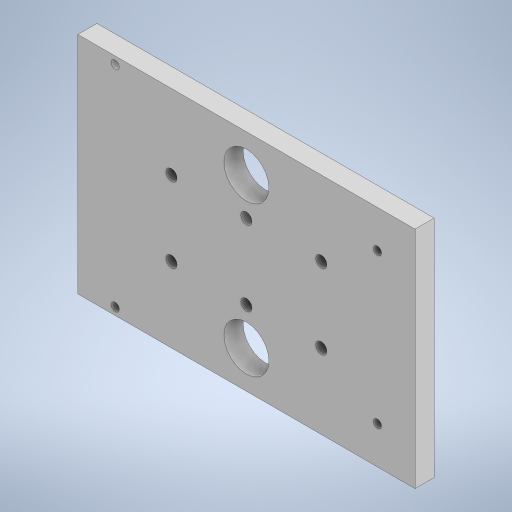
# Autodesk Inventor part: lidar mounting plate
Saved by Autodesk Inventor 2023.2 (Build 272271000, 271)
## iProperties
Created: 2024-08-12
Part Number: lidar mounting plate
Material: Generic
Document SubType Name: Modeling
Designer: PC
Density: 1 g/cm^3
Appearance: Default
Author: PC
Autodesk Inventor part; units mm, degrees
ref_plane "YZ Plane" through (0, 0, 0) normal (1, 0, 0) x (0, 1, 0)
ref_plane "XZ Plane" through (0, 0, 0) normal (0, 1, 0) x (-1, 0, 0)
ref_plane "XY Plane" through (0, 0, 0) normal (0, 0, 1) x (1, 0, 0)
sketch "Sketch1" plane through (0, 0, 0) normal (0, 0, 1) x (1, 0, 0)
  line L0 (-45, -30) -> (45, -30)
  line L1 (45, -30) -> (45, 30)
  line L2 (45, 30) -> (-45, 30)
  line L3 (-45, 30) -> (-45, -30)
  line L4 (-45, -30) -> (45, 30) construction
  line L5 (45, -30) -> (-45, 30) construction
  circle A0 centre (-35, -28) radius 1.092
  circle A1 centre (35, -20) radius 1.092
  line L6 (0, 0) -> (14.1537, 0) construction
  circle A2 centre (-35, 28) radius 1.092
  circle A3 centre (35, 20) radius 1.092
  circle A4 centre (-20, 10) radius 1.5
  circle A5 centre (0, 10) radius 1.5
  circle A6 centre (20, 10) radius 1.5
  circle A7 centre (-20, -10) radius 1.5
  circle A8 centre (0, -10) radius 1.5
  circle A9 centre (20, -10) radius 1.5
  circle A10 centre (0, 20) radius 6
  circle A11 centre (0, -20) radius 6
  dimension "d0" = 90
  dimension "d1" = 60
  dimension "d7" = 2.184
  dimension "d8" = 2.184
  dimension "d11" = 2
  dimension "d19" = 70
  dimension "d22" = 10
  dimension "d23" = 10
  dimension "d24" = 3
  dimension "d25" = 3
  dimension "d26" = 3
  dimension "d27" = 3
  dimension "d28" = 3
  dimension "d29" = 3
  dimension "d30" = 10
  dimension "d31" = 10
  dimension "d32" = 20
  dimension "d33" = 20
  dimension "d34" = 12
  dimension "d35" = 12
  dimension "d36" = 20
  dimension "d37" = 20
  constraints: 14 end point, 12 centre point, 6 vertical alignment, 4 horizontal alignment, 2 horizontal, 2 midpoint, 2 parallel, 2 symmetric about line, 1 perpendicular, 2 other
  measures "d0" distance of L2.end L1.end
  measures "d1" distance of L1.end L0.end
  measures "d7" diameter of A0
  measures "d8" diameter of A1
  measures "d11" distance from line of L0 A0.centre
  measures "d19" horizontal distance of A1.centre A0.centre
  measures "d22" distance from line of L0 A1.centre
  measures "d23" distance from line of L3 A0.centre
  measures "d24" diameter of A4
  measures "d25" diameter of A5
  measures "d26" diameter of A6
  measures "d27" diameter of A7
  measures "d28" diameter of A8
  measures "d29" diameter of A9
  measures "d30" vertical distance of L6.start A4.centre
  measures "d31" vertical distance of L6.start A7.centre
  measures "d32" horizontal distance of L6.start A4.centre
  measures "d33" horizontal distance of A6.centre L6.start
  measures "d34" diameter of A10
  measures "d35" diameter of A11
  measures "d36" distance of L6.start A10.centre
  measures "d37" distance of L6.start A11.centre
extrude "Extrusion1" add sketch "Sketch1" along normal blind 5.1
body "Solid1"
